Autodesk Fusion 360 part; units mm, degrees
(part 2 of 3)
sketch "Sketch15" plane through (0, 3, 0) normal (0, 1, 0) x (-1, 0, 0)
  line L0 (-66.9, 56.225) -> (-66.9, 85.865)
  line L1 (-66.9, 85.865) -> (-48.98, 85.865)
  line L2 (-48.98, 85.865) -> (-48.98, 56.225)
  line L3 (-48.98, 56.225) -> (-66.9, 56.225)
  line L4 (-83.08, 18.85) -> (0, 18.85)
  line L5 (0, 18.85) -> (0, 100)
  line L6 (0, 100) -> (-83.08, 100)
  line L7 (-83.08, 100) -> (-83.08, 18.85)
  line L8 (-38.05, 42.9) -> (-38.05, 56.9)
  line L9 (-38.05, 56.9) -> (-24.05, 56.9)
  line L10 (-24.05, 56.9) -> (-24.05, 42.9)
  line L11 (-24.05, 42.9) -> (-38.05, 42.9)
  line L12 (-19, 23.85) -> (-19, 37.85)
  line L13 (-19, 37.85) -> (-5, 37.85)
  line L14 (-5, 37.85) -> (-5, 23.85)
  line L15 (-5, 23.85) -> (-19, 23.85)
  line L16 (-19, 56.9) -> (-5, 56.9)
  line L17 (-5, 56.9) -> (-5, 42.9)
  line L18 (-5, 42.9) -> (-19, 42.9)
  line L19 (-19, 42.9) -> (-19, 56.9)
  line L20 (-38.05, 75.95) -> (-24.05, 75.95)
  line L21 (-24.05, 75.95) -> (-24.05, 61.95)
  line L22 (-24.05, 61.95) -> (-38.05, 61.95)
  line L23 (-38.05, 61.95) -> (-38.05, 75.95)
  line L24 (-19, 95) -> (-5, 95)
  line L25 (-5, 95) -> (-5, 81)
  line L26 (-5, 81) -> (-19, 81)
  line L27 (-19, 81) -> (-19, 95)
  line L28 (-38.05, 23.85) -> (-38.05, 37.85)
  line L29 (-38.05, 37.85) -> (-24.05, 37.85)
  line L30 (-24.05, 37.85) -> (-24.05, 23.85)
  line L31 (-24.05, 23.85) -> (-38.05, 23.85)
  line L32 (-19, 61.95) -> (-19, 75.95)
  line L33 (-19, 75.95) -> (-5, 75.95)
  line L34 (-5, 75.95) -> (-5, 61.95)
  line L35 (-5, 61.95) -> (-19, 61.95)
  line L36 (-38.05, 95) -> (-24.05, 95)
  line L37 (-24.05, 95) -> (-24.05, 81)
  line L38 (-24.05, 81) -> (-38.05, 81)
  line L39 (-38.05, 81) -> (-38.05, 95)
  circle A0 centre (-80.08, 97.0008) radius 1.5
  circle A1 centre (-2.9851, 97) radius 1.5
  circle A2 centre (-80.08, 21.85) radius 1.5
  circle A3 centre (-2.9679, 21.85) radius 1.5
  circle A4 centre (-60.755, 38.6) radius 4.5
extrude "Extrude26" add sketch "Sketch15" against normal blind 3 contours A0 | A1 | A2 | A3
sketch "Sketch16" plane through (0, 3, 0) normal (0, 1, 0) x (-1, 0, 0)
  line L0 (-66.9, 56.225) -> (-66.9, 85.865)
  line L1 (-66.9, 85.865) -> (-48.98, 85.865)
  line L2 (-48.98, 85.865) -> (-48.98, 56.225)
  line L3 (-48.98, 56.225) -> (-66.9, 56.225)
  line L4 (-83.08, 18.85) -> (0, 18.85)
  line L5 (0, 18.85) -> (0, 100)
  line L6 (0, 100) -> (-83.08, 100)
  line L7 (-83.08, 100) -> (-83.08, 18.85)
  line L8 (-38.05, 42.9) -> (-38.05, 56.9)
  line L9 (-38.05, 56.9) -> (-24.05, 56.9)
  line L10 (-24.05, 56.9) -> (-24.05, 42.9)
  line L11 (-24.05, 42.9) -> (-38.05, 42.9)
  line L12 (-19, 23.85) -> (-19, 37.85)
  line L13 (-19, 37.85) -> (-5, 37.85)
  line L14 (-5, 37.85) -> (-5, 23.85)
  line L15 (-5, 23.85) -> (-19, 23.85)
  line L16 (-19, 56.9) -> (-5, 56.9)
  line L17 (-5, 56.9) -> (-5, 42.9)
  line L18 (-5, 42.9) -> (-19, 42.9)
  line L19 (-19, 42.9) -> (-19, 56.9)
  line L20 (-38.05, 75.95) -> (-24.05, 75.95)
  line L21 (-24.05, 75.95) -> (-24.05, 61.95)
  line L22 (-24.05, 61.95) -> (-38.05, 61.95)
  line L23 (-38.05, 61.95) -> (-38.05, 75.95)
  line L24 (-19, 95) -> (-5, 95)
  line L25 (-5, 95) -> (-5, 81)
  line L26 (-5, 81) -> (-19, 81)
  line L27 (-19, 81) -> (-19, 95)
  line L28 (-38.05, 23.85) -> (-38.05, 37.85)
  line L29 (-38.05, 37.85) -> (-24.05, 37.85)
  line L30 (-24.05, 37.85) -> (-24.05, 23.85)
  line L31 (-24.05, 23.85) -> (-38.05, 23.85)
  line L32 (-19, 61.95) -> (-19, 75.95)
  line L33 (-19, 75.95) -> (-5, 75.95)
  line L34 (-5, 75.95) -> (-5, 61.95)
  line L35 (-5, 61.95) -> (-19, 61.95)
  line L36 (-38.05, 95) -> (-24.05, 95)
  line L37 (-24.05, 95) -> (-24.05, 81)
  line L38 (-24.05, 81) -> (-38.05, 81)
  line L39 (-38.05, 81) -> (-38.05, 95)
  circle A0 centre (-60.755, 38.6) radius 4.5
  line L40 (0, 21.368) -> (-2.5, 21.368)
  line L41 (-2.5, 21.368) -> (-2.5, 18.868)
  line L42 (-80.5906, 18.85) -> (-80.5906, 21.35)
  line L43 (-80.5906, 21.35) -> (-83.0906, 21.35)
  line L44 (-83.08, 97.4836) -> (-80.58, 97.4836)
  line L45 (-80.58, 97.4836) -> (-80.58, 99.9836)
  line L46 (0, 97.4763) -> (-2.5, 97.4763)
  line L47 (-2.5, 97.4763) -> (-2.5, 99.9763)
  circle A1 centre (-2.5, 97.4763) radius 1
  circle A2 centre (-80.58, 97.4836) radius 1
  circle A3 centre (-80.5906, 21.35) radius 1
  circle A4 centre (-2.5, 21.368) radius 1
  dimension "d162" = 2.5
  dimension "d163" = 2.5
  dimension "d164" = 2.5
  dimension "d165" = 2.5
  dimension "d166" = 2.5
  dimension "d167" = 2.5
  dimension "d168" = 2.5
  dimension "d169" = 2.5
  dimension "d170" = 2
  dimension "d171" = 2
  dimension "d172" = 2
  dimension "d173" = 2
  constraint coincident L5 L40.start
  constraint perpendicular L5 L40
  constraint perpendicular L40 L41
  constraint coincident L4 L42.start
  constraint perpendicular L4 L42
  constraint perpendicular L42 L43
  constraint coincident L7 L44.start
  constraint perpendicular L7 L44
  constraint perpendicular L44 L45
  constraint coincident L5 L46.start
  constraint perpendicular L5 L46
  constraint perpendicular L46 L47
  constraint coincident L46.end L47.start
  constraint coincident L44.end L45.start
  constraint coincident L42.end L43.start
  constraint coincident L40.end L41.start
  measures "d162" distance of L40.start L40.end
  measures "d163" distance of L40.end L41.end
  measures "d164" distance of L42.start L42.end
  measures "d165" distance of L42.end L43.end
  measures "d166" distance of L44.start L44.end
  measures "d167" distance of L44.end L45.end
  measures "d168" distance of L46.start L46.end
  measures "d169" distance of L46.end L47.end
  measures "d170" diameter of A1
  measures "d171" diameter of A2
  measures "d172" diameter of A3
  measures "d173" diameter of A4
extrude "Extrude27" cut sketch "Sketch16" against normal blind 5.5 contours L42 L43 A3 | L42 L43 A3 | L40 L41 A4 | L40 L41 A4 | L44 L45 A2 | L44 L45 A2 | L46 L47 A1 | L46 L47 A1
extrude "Extrude28" cut 4 faces at (44.9701, -4, 27.857) (77.0768, -4, 30.8265) (76.1742, -4, 90.9914) (44.34, -4, 90.7407) along direction (0, 1, 0) blind 0.5
extrude "Extrude29" cut 1 faces at (76.5447, 3, 58.3529) along direction (0, -1, 0) blind 1
extrude "Extrude30" cut 4 faces at (44.34, -3.5, 90.7407) (76.1742, -3.5, 90.9914) (77.0768, -3.5, 30.8265) (44.9701, -3.5, 27.857) along direction (0, 1, 0) blind 1
sketch "Sketch17" plane through (0, 2, 0) normal (0, 1, 0) x (-1, 0, 0)
  circle A0 centre (-80.5906, 21.35) radius 1
  circle A1 centre (-80.58, 97.4836) radius 1
  circle A2 centre (-2.5, 21.368) radius 1
  circle A3 centre (-2.5, 97.4763) radius 1
  line L0 (-66.9, 56.225) -> (-66.9, 85.865)
  line L1 (-66.9, 85.865) -> (-48.98, 85.865)
  line L2 (-48.98, 85.865) -> (-48.98, 56.225)
  line L3 (-48.98, 56.225) -> (-66.9, 56.225)
  line L4 (-83.08, 18.85) -> (0, 18.85)
  line L5 (0, 18.85) -> (0, 100)
  line L6 (0, 100) -> (-83.08, 100)
  line L7 (-83.08, 100) -> (-83.08, 18.85)
  line L8 (-38.05, 42.9) -> (-38.05, 56.9)
  line L9 (-38.05, 56.9) -> (-24.05, 56.9)
  line L10 (-24.05, 56.9) -> (-24.05, 42.9)
  line L11 (-24.05, 42.9) -> (-38.05, 42.9)
  line L12 (-19, 23.85) -> (-19, 37.85)
  line L13 (-19, 37.85) -> (-5, 37.85)
  line L14 (-5, 37.85) -> (-5, 23.85)
  line L15 (-5, 23.85) -> (-19, 23.85)
  line L16 (-19, 56.9) -> (-5, 56.9)
  line L17 (-5, 56.9) -> (-5, 42.9)
  line L18 (-5, 42.9) -> (-19, 42.9)
  line L19 (-19, 42.9) -> (-19, 56.9)
  line L20 (-38.05, 75.95) -> (-24.05, 75.95)
  line L21 (-24.05, 75.95) -> (-24.05, 61.95)
  line L22 (-24.05, 61.95) -> (-38.05, 61.95)
  line L23 (-38.05, 61.95) -> (-38.05, 75.95)
  line L24 (-19, 95) -> (-5, 95)
  line L25 (-5, 95) -> (-5, 81)
  line L26 (-5, 81) -> (-19, 81)
  line L27 (-19, 81) -> (-19, 95)
  line L28 (-38.05, 23.85) -> (-38.05, 37.85)
  line L29 (-38.05, 37.85) -> (-24.05, 37.85)
  line L30 (-24.05, 37.85) -> (-24.05, 23.85)
  line L31 (-24.05, 23.85) -> (-38.05, 23.85)
  line L32 (-19, 61.95) -> (-19, 75.95)
  line L33 (-19, 75.95) -> (-5, 75.95)
  line L34 (-5, 75.95) -> (-5, 61.95)
  line L35 (-5, 61.95) -> (-19, 61.95)
  line L36 (-38.05, 95) -> (-24.05, 95)
  line L37 (-24.05, 95) -> (-24.05, 81)
  line L38 (-24.05, 81) -> (-38.05, 81)
  line L39 (-38.05, 81) -> (-38.05, 95)
  circle A4 centre (-45.8889, 88.9935) radius 2
  circle A5 centre (-45.9348, 29.975) radius 2
  circle A6 centre (-75.1, 88.9) radius 2
  circle A7 centre (-74.9, 29.9) radius 2
  line L40 (-54.755, 44.6) -> (-54.755, 32.6)
  line L41 (-54.755, 32.6) -> (-66.755, 32.6)
  line L42 (-66.755, 32.6) -> (-66.755, 44.6)
  line L43 (-66.755, 44.6) -> (-54.755, 44.6)
extrude "Extrude31" add sketch "Sketch17" against normal blind 0.5 contours A4 | A5 | A6 | A7
sketch "Sketch18" plane through (0, 2, 0) normal (0, 1, 0) x (-1, 0, 0)
  circle A0 centre (-80.5906, 21.35) radius 1
  circle A1 centre (-80.58, 97.4836) radius 1
  circle A2 centre (-2.5, 21.368) radius 1
  circle A3 centre (-2.5, 97.4763) radius 1
  line L0 (-66.9, 56.225) -> (-66.9, 85.865)
  line L1 (-66.9, 85.865) -> (-48.98, 85.865)
  line L2 (-48.98, 85.865) -> (-48.98, 56.225)
  line L3 (-48.98, 56.225) -> (-66.9, 56.225)
  line L4 (-83.08, 18.85) -> (0, 18.85)
  line L5 (0, 18.85) -> (0, 100)
  line L6 (0, 100) -> (-83.08, 100)
  line L7 (-83.08, 100) -> (-83.08, 18.85)
  line L8 (-38.05, 42.9) -> (-38.05, 56.9)
  line L9 (-38.05, 56.9) -> (-24.05, 56.9)
  line L10 (-24.05, 56.9) -> (-24.05, 42.9)
  line L11 (-24.05, 42.9) -> (-38.05, 42.9)
  line L12 (-19, 23.85) -> (-19, 37.85)
  line L13 (-19, 37.85) -> (-5, 37.85)
  line L14 (-5, 37.85) -> (-5, 23.85)
  line L15 (-5, 23.85) -> (-19, 23.85)
  line L16 (-19, 56.9) -> (-5, 56.9)
  line L17 (-5, 56.9) -> (-5, 42.9)
  line L18 (-5, 42.9) -> (-19, 42.9)
  line L19 (-19, 42.9) -> (-19, 56.9)
  line L20 (-38.05, 75.95) -> (-24.05, 75.95)
  line L21 (-24.05, 75.95) -> (-24.05, 61.95)
  line L22 (-24.05, 61.95) -> (-38.05, 61.95)
  line L23 (-38.05, 61.95) -> (-38.05, 75.95)
  line L24 (-19, 95) -> (-5, 95)
  line L25 (-5, 95) -> (-5, 81)
  line L26 (-5, 81) -> (-19, 81)
  line L27 (-19, 81) -> (-19, 95)
  line L28 (-38.05, 23.85) -> (-38.05, 37.85)
  line L29 (-38.05, 37.85) -> (-24.05, 37.85)
  line L30 (-24.05, 37.85) -> (-24.05, 23.85)
  line L31 (-24.05, 23.85) -> (-38.05, 23.85)
  line L32 (-19, 61.95) -> (-19, 75.95)
  line L33 (-19, 75.95) -> (-5, 75.95)
  line L34 (-5, 75.95) -> (-5, 61.95)
  line L35 (-5, 61.95) -> (-19, 61.95)
  line L36 (-38.05, 95) -> (-24.05, 95)
  line L37 (-24.05, 95) -> (-24.05, 81)
  line L38 (-24.05, 81) -> (-38.05, 81)
  line L39 (-38.05, 81) -> (-38.05, 95)
  line L40 (-54.755, 44.6) -> (-54.755, 32.6)
  line L41 (-54.755, 32.6) -> (-66.755, 32.6)
  line L42 (-66.755, 32.6) -> (-66.755, 44.6)
  line L43 (-66.755, 44.6) -> (-54.755, 44.6)
extrude "Extrude32" add sketch "Sketch18" against normal blind 0.5 contours L40 L41 L42 L43
sketch "Sketch19" plane through (0, 1.5, 0) normal (0, -1, 0) x (1, 0, 0)
  line L0 (66.755, 32.6) -> (66.755, 44.6)
  line L1 (66.755, 44.6) -> (54.755, 44.6)
  line L2 (54.755, 44.6) -> (54.755, 32.6)
  line L3 (54.755, 32.6) -> (66.755, 32.6)
  circle A0 centre (60.7672, 38.6189) radius 6
  dimension "d186" = 12
  measures "d186" diameter of A0
extrude "Extrude33" cut sketch "Sketch19" against normal blind 1 contours L0 L1 A0 picked at (62.3334, 39.4206)
sketch "Sketch20" plane through (0, 0, 0) normal (0, -1, 0) x (1, 0, 0)
  line L0 (66.9, 85.865) -> (66.9, 56.225)
  line L1 (66.9, 56.225) -> (48.98, 56.225)
  line L2 (48.98, 56.225) -> (48.98, 85.7386)
  arc A0 (49.1082, 85.865) -> (48.98, 85.7386) centre (45.8848, 89.005) ccw
  line L3 (49.1082, 85.865) -> (66.9, 85.865)
  circle A1 centre (75.1296, 88.925) radius 4.5
  circle A2 centre (45.9348, 29.975) radius 4.5
  line L4 (83.08, 100) -> (0, 100)
  line L5 (0, 100) -> (0, 18.85)
  line L6 (0, 18.85) -> (83.08, 18.85)
  line L7 (83.08, 18.85) -> (83.08, 100)
  line L8 (24.05, 95) -> (38.05, 95)
  line L9 (38.05, 95) -> (38.05, 81)
  line L10 (38.05, 81) -> (24.05, 81)
  line L11 (24.05, 81) -> (24.05, 95)
  line L12 (19, 75.95) -> (19, 61.95)
  line L13 (19, 61.95) -> (5, 61.95)
  line L14 (5, 61.95) -> (5, 75.95)
  line L15 (5, 75.95) -> (19, 75.95)
  line L16 (38.05, 37.85) -> (38.05, 23.85)
  line L17 (38.05, 23.85) -> (24.05, 23.85)
  line L18 (24.05, 23.85) -> (24.05, 37.85)
  line L19 (24.05, 37.85) -> (38.05, 37.85)
  line L20 (5, 95) -> (19, 95)
  line L21 (19, 95) -> (19, 81)
  line L22 (19, 81) -> (5, 81)
  line L23 (5, 81) -> (5, 95)
  line L24 (24.05, 75.95) -> (38.05, 75.95)
  line L25 (38.05, 75.95) -> (38.05, 61.95)
  line L26 (38.05, 61.95) -> (24.05, 61.95)
  line L27 (24.05, 61.95) -> (24.05, 75.95)
  line L28 (5, 56.9) -> (19, 56.9)
  line L29 (19, 56.9) -> (19, 42.9)
  line L30 (19, 42.9) -> (5, 42.9)
  line L31 (5, 42.9) -> (5, 56.9)
  line L32 (19, 37.85) -> (19, 23.85)
  line L33 (19, 23.85) -> (5, 23.85)
  line L34 (5, 23.85) -> (5, 37.85)
  line L35 (5, 37.85) -> (19, 37.85)
  line L36 (38.05, 56.9) -> (38.05, 42.9)
  line L37 (38.05, 42.9) -> (24.05, 42.9)
  line L38 (24.05, 42.9) -> (24.05, 56.9)
  line L39 (24.05, 56.9) -> (38.05, 56.9)
  line L40 (54.755, 44.6) -> (66.755, 44.6)
  line L41 (66.755, 44.6) -> (66.755, 32.6)
  line L42 (66.755, 32.6) -> (54.755, 32.6)
  line L43 (54.755, 32.6) -> (54.755, 44.6)
  circle A3 centre (74.9435, 29.945) radius 4.5
  circle A4 centre (2.5, 97.4763) radius 1
  circle A5 centre (2.5, 21.368) radius 1
  circle A6 centre (80.58, 97.4836) radius 1
  circle A7 centre (80.5906, 21.35) radius 1
extrude "Extrude34" add sketch "Sketch20" against normal blind 2 contours A4 | A5 | A6 | A7
sketch "Sketch21" plane through (0, 0, 0) normal (0, -1, 0) x (1, 0, 0)
  line L0 (66.9, 85.865) -> (66.9, 56.225)
  line L1 (66.9, 56.225) -> (48.98, 56.225)
  line L2 (48.98, 56.225) -> (48.98, 85.7386)
  arc A0 (49.1082, 85.865) -> (48.98, 85.7386) centre (45.8848, 89.005) ccw
  line L3 (49.1082, 85.865) -> (66.9, 85.865)
  circle A1 centre (75.1296, 88.925) radius 4.5
  circle A2 centre (45.9348, 29.975) radius 4.5
  line L4 (83.08, 100) -> (0, 100)
  line L5 (0, 100) -> (0, 18.85)
  line L6 (0, 18.85) -> (83.08, 18.85)
  line L7 (83.08, 18.85) -> (83.08, 100)
  line L8 (24.05, 95) -> (38.05, 95)
  line L9 (38.05, 95) -> (38.05, 81)
  line L10 (38.05, 81) -> (24.05, 81)
  line L11 (24.05, 81) -> (24.05, 95)
  line L12 (19, 75.95) -> (19, 61.95)
  line L13 (19, 61.95) -> (5, 61.95)
  line L14 (5, 61.95) -> (5, 75.95)
  line L15 (5, 75.95) -> (19, 75.95)
  line L16 (38.05, 37.85) -> (38.05, 23.85)
  line L17 (38.05, 23.85) -> (24.05, 23.85)
  line L18 (24.05, 23.85) -> (24.05, 37.85)
  line L19 (24.05, 37.85) -> (38.05, 37.85)
  line L20 (5, 95) -> (19, 95)
  line L21 (19, 95) -> (19, 81)
  line L22 (19, 81) -> (5, 81)
  line L23 (5, 81) -> (5, 95)
  line L24 (24.05, 75.95) -> (38.05, 75.95)
  line L25 (38.05, 75.95) -> (38.05, 61.95)
  line L26 (38.05, 61.95) -> (24.05, 61.95)
  line L27 (24.05, 61.95) -> (24.05, 75.95)
  line L28 (5, 56.9) -> (19, 56.9)
  line L29 (19, 56.9) -> (19, 42.9)
  line L30 (19, 42.9) -> (5, 42.9)
  line L31 (5, 42.9) -> (5, 56.9)
  line L32 (19, 37.85) -> (19, 23.85)
  line L33 (19, 23.85) -> (5, 23.85)
  line L34 (5, 23.85) -> (5, 37.85)
  line L35 (5, 37.85) -> (19, 37.85)
  line L36 (38.05, 56.9) -> (38.05, 42.9)
  line L37 (38.05, 42.9) -> (24.05, 42.9)
  line L38 (24.05, 42.9) -> (24.05, 56.9)
  line L39 (24.05, 56.9) -> (38.05, 56.9)
  line L40 (54.755, 44.6) -> (66.755, 44.6)
  line L41 (66.755, 44.6) -> (66.755, 32.6)
  line L42 (66.755, 32.6) -> (54.755, 32.6)
  line L43 (54.755, 32.6) -> (54.755, 44.6)
  circle A3 centre (74.9435, 29.945) radius 4.5
  circle A4 centre (3.9673, 22.8373) radius 4
  circle A5 centre (3.9951, 96.0403) radius 4
  circle A6 centre (79.0997, 96.034) radius 4
  circle A7 centre (79.1068, 22.8281) radius 4
  dimension "d191" = 8
  dimension "d192" = 5.625
  dimension "d193" = 8
  dimension "d194" = 8
  dimension "d195" = 8
  measures "d191" diameter of A4
  measures "d192" distance of L4.end A5.centre
  measures "d193" diameter of A5
  measures "d194" diameter of A6
  measures "d195" diameter of A7
extrude "Extrude35" cut sketch "Sketch21" against normal blind 3 contours L4 L7 A6 | L6 L7 A7 | L4 L5 A5 | L5 L6 A4
extrude "Extrude36" cut 2 faces at (65.3995, 1.5, 43.6074) (55.9645, 1.5, 33.7699) along direction (0, 1, 0) blind 0.1
sketch "Sketch22" plane through (0, 0, 0) normal (0, -1, 0) x (1, 0, 0)
  arc A0 (0, 22.3271) -> (3.6486, 18.85) centre (3.9673, 22.8373) ccw
  line L0 (3.6486, 18.85) -> (79.525, 18.85)
  arc A1 (79.525, 18.85) -> (83.08, 22.3661) centre (79.1068, 22.8281) ccw
  line L1 (83.08, 22.3661) -> (83.08, 96.4304)
  arc A2 (83.08, 96.4304) -> (79.62, 100) centre (79.0997, 96.034) ccw
  line L2 (79.62, 100) -> (3.429, 100)
  arc A3 (3.429, 100) -> (0, 96.2373) centre (3.9951, 96.0403) ccw
  line L3 (0, 96.2373) -> (0, 22.3271)
  circle A4 centre (74.9435, 29.945) radius 4.5
  line L4 (54.755, 44.6) -> (66.755, 44.6)
  line L5 (66.755, 44.6) -> (66.755, 32.6)
  line L6 (66.755, 32.6) -> (54.755, 32.6)
  line L7 (54.755, 32.6) -> (54.755, 44.6)
  line L8 (38.05, 56.9) -> (38.05, 42.9)
  line L9 (38.05, 42.9) -> (24.05, 42.9)
  line L10 (24.05, 42.9) -> (24.05, 56.9)
  line L11 (24.05, 56.9) -> (38.05, 56.9)
  line L12 (19, 37.85) -> (19, 23.85)
  line L13 (19, 23.85) -> (5, 23.85)
  line L14 (5, 23.85) -> (5, 37.85)
  line L15 (5, 37.85) -> (19, 37.85)
  line L16 (5, 56.9) -> (19, 56.9)
  line L17 (19, 56.9) -> (19, 42.9)
  line L18 (19, 42.9) -> (5, 42.9)
  line L19 (5, 42.9) -> (5, 56.9)
  line L20 (24.05, 75.95) -> (38.05, 75.95)
  line L21 (38.05, 75.95) -> (38.05, 61.95)
  line L22 (38.05, 61.95) -> (24.05, 61.95)
  line L23 (24.05, 61.95) -> (24.05, 75.95)
  line L24 (5, 95) -> (19, 95)
  line L25 (19, 95) -> (19, 81)
  line L26 (19, 81) -> (5, 81)
  line L27 (5, 81) -> (5, 95)
  line L28 (38.05, 37.85) -> (38.05, 23.85)
  line L29 (38.05, 23.85) -> (24.05, 23.85)
  line L30 (24.05, 23.85) -> (24.05, 37.85)
  line L31 (24.05, 37.85) -> (38.05, 37.85)
  line L32 (19, 75.95) -> (19, 61.95)
  line L33 (19, 61.95) -> (5, 61.95)
  line L34 (5, 61.95) -> (5, 75.95)
  line L35 (5, 75.95) -> (19, 75.95)
  line L36 (24.05, 95) -> (38.05, 95)
  line L37 (38.05, 95) -> (38.05, 81)
  line L38 (38.05, 81) -> (24.05, 81)
  line L39 (24.05, 81) -> (24.05, 95)
  circle A5 centre (45.9348, 29.975) radius 4.5
  circle A6 centre (75.1296, 88.925) radius 4.5
  line L40 (66.9, 85.865) -> (66.9, 56.225)
  line L41 (66.9, 56.225) -> (48.98, 56.225)
  line L42 (48.98, 56.225) -> (48.98, 85.7386)
  arc A7 (49.1082, 85.865) -> (48.98, 85.7386) centre (45.8848, 89.005) ccw
  line L43 (49.1082, 85.865) -> (66.9, 85.865)
  circle A8 centre (3, 97) radius 1.75
  circle A9 centre (3, 97) radius 1
  line L44 (3, 97) -> (3, 100)
  line L45 (3, 97) -> (0, 97)
  line L46 (80.0899, 100) -> (80.0899, 97)
  line L47 (80.0899, 97) -> (83.0899, 97)
  circle A10 centre (80.0899, 97) radius 1
  line L48 (83.0763, 21.8589) -> (80.0763, 21.8589)
  line L49 (80.0763, 21.8589) -> (80.0763, 18.8589)
  circle A11 centre (80.0763, 21.8589) radius 1
  line L50 (-0.0037, 21.8321) -> (2.9963, 21.8321)
  line L51 (2.9963, 21.8321) -> (2.9963, 18.8321)
  circle A12 centre (2.9963, 21.8321) radius 1
  dimension "d200" = 3.5
  dimension "d201" = 2
  dimension "d202" = 3
  dimension "d203" = 3
  dimension "d204" = 2
  dimension "d205" = 3
  dimension "d206" = 3
  dimension "d207" = 2
  dimension "d208" = 3
  dimension "d209" = 3
  dimension "d210" = 2
  constraint concentric A8 A9
  constraint coincident A8.centre A9.centre
  constraint vertical L44
  constraint horizontal L45
  constraint vertical L46
  constraint perpendicular L1 L47
  constraint coincident L46.end L47.start
  constraint horizontal L48
  constraint perpendicular L48 L49
  constraint coincident L48.end L49.start
  constraint horizontal L50
  constraint perpendicular L50 L51
  constraint coincident L50.end L51.start
  measures "d200" diameter of A8
  measures "d201" diameter of A9
  measures "d202" distance of L46.start L46.end
  measures "d203" distance of L46.end L47.end
  measures "d204" diameter of A10
  measures "d205" distance of L48.start L48.end
  measures "d206" distance of L48.end L49.end
  measures "d207" diameter of A11
  measures "d208" distance of L50.start L50.end
  measures "d209" distance of L50.end L51.end
  measures "d210" diameter of A12
extrude "Extrude37" cut sketch "Sketch22" against normal blind 7 contours L50 L51 A12 | L50 L51 A12 | A9 L44 L45 | A9 L44 L45 | L48 L49 A11 | L48 L49 A11 | L46 L47 A10 | L46 L47 A10
sketch "Sketch23" plane through (0, 0, 0) normal (0, -1, 0) x (1, 0, 0)
  line L0 (66.9, 85.865) -> (66.9, 56.225)
  line L1 (66.9, 56.225) -> (48.98, 56.225)
  line L2 (48.98, 56.225) -> (48.98, 85.7386)
  arc A0 (49.1082, 85.865) -> (48.98, 85.7386) centre (45.8848, 89.005) ccw
  line L3 (49.1082, 85.865) -> (66.9, 85.865)
  circle A1 centre (75.1296, 88.925) radius 4.5
  circle A2 centre (45.9348, 29.975) radius 4.5
  line L4 (24.05, 95) -> (38.05, 95)
  line L5 (38.05, 95) -> (38.05, 81)
  line L6 (38.05, 81) -> (24.05, 81)
  line L7 (24.05, 81) -> (24.05, 95)
  line L8 (19, 75.95) -> (19, 61.95)
  line L9 (19, 61.95) -> (5, 61.95)
  line L10 (5, 61.95) -> (5, 75.95)
  line L11 (5, 75.95) -> (19, 75.95)
  line L12 (38.05, 37.85) -> (38.05, 23.85)
  line L13 (38.05, 23.85) -> (24.05, 23.85)
  line L14 (24.05, 23.85) -> (24.05, 37.85)
  line L15 (24.05, 37.85) -> (38.05, 37.85)
  line L16 (5, 95) -> (19, 95)
  line L17 (19, 95) -> (19, 81)
  line L18 (19, 81) -> (5, 81)
  line L19 (5, 81) -> (5, 95)
  line L20 (24.05, 75.95) -> (38.05, 75.95)
  line L21 (38.05, 75.95) -> (38.05, 61.95)
  line L22 (38.05, 61.95) -> (24.05, 61.95)
  line L23 (24.05, 61.95) -> (24.05, 75.95)
  line L24 (5, 56.9) -> (19, 56.9)
  line L25 (19, 56.9) -> (19, 42.9)
  line L26 (19, 42.9) -> (5, 42.9)
  line L27 (5, 42.9) -> (5, 56.9)
  line L28 (19, 37.85) -> (19, 23.85)
  line L29 (19, 23.85) -> (5, 23.85)
  line L30 (5, 23.85) -> (5, 37.85)
  line L31 (5, 37.85) -> (19, 37.85)
  line L32 (38.05, 56.9) -> (38.05, 42.9)
  line L33 (38.05, 42.9) -> (24.05, 42.9)
  line L34 (24.05, 42.9) -> (24.05, 56.9)
  line L35 (24.05, 56.9) -> (38.05, 56.9)
  line L36 (54.755, 44.6) -> (66.755, 44.6)
  line L37 (66.755, 44.6) -> (66.755, 32.6)
  line L38 (66.755, 32.6) -> (54.755, 32.6)
  line L39 (54.755, 32.6) -> (54.755, 44.6)
  circle A3 centre (74.9435, 29.945) radius 4.5
  arc A4 (0, 22.3271) -> (3.6486, 18.85) centre (3.9673, 22.8373) ccw
  line L40 (3.6486, 18.85) -> (79.525, 18.85)
  arc A5 (79.525, 18.85) -> (83.08, 22.3661) centre (79.1068, 22.8281) ccw
  line L41 (83.08, 22.3661) -> (83.08, 96.4304)
  arc A6 (83.08, 96.4304) -> (79.62, 100) centre (79.0997, 96.034) ccw
  line L42 (79.62, 100) -> (3.429, 100)
  arc A7 (3.429, 100) -> (0, 96.2373) centre (3.9951, 96.0403) ccw
  line L43 (0, 96.2373) -> (0, 22.3271)
  circle A8 centre (80.0763, 21.8589) radius 1
  circle A9 centre (2.9963, 21.8321) radius 1
  circle A10 centre (80.0899, 97) radius 1
  circle A11 centre (3, 97) radius 1
sketch "Sketch24" plane through (0, 2, 0) normal (0, 1, 0) x (-1, 0, 0)
  line L0 (-38.05, 95) -> (-24.05, 95)
  line L1 (-24.05, 95) -> (-24.05, 81)
  line L2 (-24.05, 81) -> (-38.05, 81)
  line L3 (-38.05, 81) -> (-38.05, 95)
  line L4 (-19, 61.95) -> (-19, 75.95)
  line L5 (-19, 75.95) -> (-5, 75.95)
  line L6 (-5, 75.95) -> (-5, 61.95)
  line L7 (-5, 61.95) -> (-19, 61.95)
  line L8 (-38.05, 23.85) -> (-38.05, 37.85)
  line L9 (-38.05, 37.85) -> (-24.05, 37.85)
  line L10 (-24.05, 37.85) -> (-24.05, 23.85)
  line L11 (-24.05, 23.85) -> (-38.05, 23.85)
  line L12 (-19, 95) -> (-5, 95)
  line L13 (-5, 95) -> (-5, 81)
  line L14 (-5, 81) -> (-19, 81)
  line L15 (-19, 81) -> (-19, 95)
  line L16 (-38.05, 75.95) -> (-24.05, 75.95)
  line L17 (-24.05, 75.95) -> (-24.05, 61.95)
  line L18 (-24.05, 61.95) -> (-38.05, 61.95)
  line L19 (-38.05, 61.95) -> (-38.05, 75.95)
  line L20 (-19, 56.9) -> (-5, 56.9)
  line L21 (-5, 56.9) -> (-5, 42.9)
  line L22 (-5, 42.9) -> (-19, 42.9)
  line L23 (-19, 42.9) -> (-19, 56.9)
  line L24 (-19, 23.85) -> (-19, 37.85)
  line L25 (-19, 37.85) -> (-5, 37.85)
  line L26 (-5, 37.85) -> (-5, 23.85)
  line L27 (-5, 23.85) -> (-19, 23.85)
  line L28 (-38.05, 42.9) -> (-38.05, 56.9)
  line L29 (-38.05, 56.9) -> (-24.05, 56.9)
  line L30 (-24.05, 56.9) -> (-24.05, 42.9)
  line L31 (-24.05, 42.9) -> (-38.05, 42.9)
  line L32 (-66.9, 56.225) -> (-66.9, 85.865)
  line L33 (-66.9, 85.865) -> (-48.98, 85.865)
  line L34 (-48.98, 85.865) -> (-48.98, 56.225)
  line L35 (-48.98, 56.225) -> (-66.9, 56.225)
  arc A0 (-61.2435, 44.6) -> (-66.755, 39.0018) centre (-60.7672, 38.6189) ccw
  line L36 (-61.2435, 44.6) -> (-60.2909, 44.6)
  arc A1 (-66.755, 38.2361) -> (-60.2909, 44.6) centre (-60.7672, 38.6189) ccw
  line L37 (-66.755, 38.2361) -> (-66.755, 39.0018)
  arc A2 (-3.6486, 18.85) -> (0, 22.3271) centre (-3.9673, 22.8373) ccw
  line L38 (0, 22.3271) -> (0, 96.2373)
  arc A3 (0, 96.2373) -> (-3.429, 100) centre (-3.9951, 96.0403) ccw
  line L39 (-3.429, 100) -> (-79.62, 100)
  arc A4 (-79.62, 100) -> (-83.08, 96.4304) centre (-79.0997, 96.034) ccw
  line L40 (-83.08, 96.4304) -> (-83.08, 22.3661)
  arc A5 (-83.08, 22.3661) -> (-79.525, 18.85) centre (-79.1068, 22.8281) ccw
  line L41 (-79.525, 18.85) -> (-3.6486, 18.85)
  circle A6 centre (-80.0763, 21.8589) radius 1
  circle A7 centre (-2.9963, 21.8321) radius 1
  circle A8 centre (-80.0899, 97) radius 1
  circle A9 centre (-3, 97) radius 1
  line L42 (-83.08, 18.85) -> (0, 18.85)
  line L43 (0, 18.85) -> (0, 100)
  line L44 (0, 100) -> (-83.08, 100)
  line L45 (-83.08, 100) -> (-83.08, 18.85)
  constraint horizontal L42
  constraint vertical L43
  constraint horizontal L44
  constraint vertical L45
delete_face "DeleteFace5" 1 faces at (81.6049, 1.3333, 99.1523)
delete_face "DeleteFace6" 1 faces at (81.7888, 1.3333, 19.8605)
extrude "Extrude38" cut 1 faces at (83.08, 0.6667, 72.95) along direction (-1, 0, 0) blind 1.93
sketch "Sketch25" plane through (0, 0, 0) normal (0, -1, 0) x (1, 0, 0)
  line L0 (81.15, 18.85) -> (81.15, 100)
  line L1 (81.15, 100) -> (3.429, 100)
  arc A0 (3.429, 100) -> (0, 96.2373) centre (3.9951, 96.0403) ccw
  line L2 (0, 96.2373) -> (0, 22.3271)
  arc A1 (0, 22.3271) -> (3.6486, 18.85) centre (3.9673, 22.8373) ccw
  line L3 (3.6486, 18.85) -> (81.15, 18.85)
  circle A2 centre (3, 97) radius 1
  circle A3 centre (80.0899, 97) radius 1
  circle A4 centre (2.9963, 21.8321) radius 1
  circle A5 centre (80.0763, 21.8589) radius 1
  circle A6 centre (74.9435, 29.945) radius 4.5
  line L4 (54.755, 44.6) -> (66.755, 44.6)
  line L5 (66.755, 44.6) -> (66.755, 32.6)
  line L6 (66.755, 32.6) -> (54.755, 32.6)
  line L7 (54.755, 32.6) -> (54.755, 44.6)
  line L8 (38.05, 56.9) -> (38.05, 42.9)
  line L9 (38.05, 42.9) -> (24.05, 42.9)
  line L10 (24.05, 42.9) -> (24.05, 56.9)
  line L11 (24.05, 56.9) -> (38.05, 56.9)
  line L12 (19, 37.85) -> (19, 23.85)
  line L13 (19, 23.85) -> (5, 23.85)
  line L14 (5, 23.85) -> (5, 37.85)
  line L15 (5, 37.85) -> (19, 37.85)
  line L16 (5, 56.9) -> (19, 56.9)
  line L17 (19, 56.9) -> (19, 42.9)
  line L18 (19, 42.9) -> (5, 42.9)
  line L19 (5, 42.9) -> (5, 56.9)
  line L20 (24.05, 75.95) -> (38.05, 75.95)
  line L21 (38.05, 75.95) -> (38.05, 61.95)
  line L22 (38.05, 61.95) -> (24.05, 61.95)
  line L23 (24.05, 61.95) -> (24.05, 75.95)
  line L24 (5, 95) -> (19, 95)
  line L25 (19, 95) -> (19, 81)
  line L26 (19, 81) -> (5, 81)
  line L27 (5, 81) -> (5, 95)
  line L28 (38.05, 37.85) -> (38.05, 23.85)
  line L29 (38.05, 23.85) -> (24.05, 23.85)
  line L30 (24.05, 23.85) -> (24.05, 37.85)
  line L31 (24.05, 37.85) -> (38.05, 37.85)
  line L32 (19, 75.95) -> (19, 61.95)
  line L33 (19, 61.95) -> (5, 61.95)
  line L34 (5, 61.95) -> (5, 75.95)
  line L35 (5, 75.95) -> (19, 75.95)
  line L36 (24.05, 95) -> (38.05, 95)
  line L37 (38.05, 95) -> (38.05, 81)
  line L38 (38.05, 81) -> (24.05, 81)
  line L39 (24.05, 81) -> (24.05, 95)
  circle A7 centre (45.9348, 29.975) radius 4.5
  circle A8 centre (75.1296, 88.925) radius 4.5
  line L40 (66.9, 85.865) -> (66.9, 56.225)
  line L41 (66.9, 56.225) -> (48.98, 56.225)
  line L42 (48.98, 56.225) -> (48.98, 85.7386)
  arc A9 (49.1082, 85.865) -> (48.98, 85.7386) centre (45.8848, 89.005) ccw
  line L43 (49.1082, 85.865) -> (66.9, 85.865)
extrude "Extrude39" add sketch "Sketch25" against normal blind 2 contours A3 | A5
sketch "Sketch26" plane through (0, 0, 0) normal (0, -1, 0) x (1, 0, 0)
  line L0 (81.15, 18.85) -> (81.15, 100)
  line L1 (81.15, 100) -> (3.429, 100)
  arc A0 (3.429, 100) -> (0, 96.2373) centre (3.9951, 96.0403) ccw
  line L2 (0, 96.2373) -> (0, 22.3271)
  arc A1 (0, 22.3271) -> (3.6486, 18.85) centre (3.9673, 22.8373) ccw
  line L3 (3.6486, 18.85) -> (81.15, 18.85)
  circle A2 centre (3, 97) radius 1
  circle A3 centre (2.9963, 21.8321) radius 1
  circle A4 centre (74.9435, 29.945) radius 4.5
  line L4 (54.755, 44.6) -> (66.755, 44.6)
  line L5 (66.755, 44.6) -> (66.755, 32.6)
  line L6 (66.755, 32.6) -> (54.755, 32.6)
  line L7 (54.755, 32.6) -> (54.755, 44.6)
  line L8 (38.05, 56.9) -> (38.05, 42.9)
  line L9 (38.05, 42.9) -> (24.05, 42.9)
  line L10 (24.05, 42.9) -> (24.05, 56.9)
  line L11 (24.05, 56.9) -> (38.05, 56.9)
  line L12 (19, 37.85) -> (19, 23.85)
  line L13 (19, 23.85) -> (5, 23.85)
  line L14 (5, 23.85) -> (5, 37.85)
  line L15 (5, 37.85) -> (19, 37.85)
  line L16 (5, 56.9) -> (19, 56.9)
  line L17 (19, 56.9) -> (19, 42.9)
  line L18 (19, 42.9) -> (5, 42.9)
  line L19 (5, 42.9) -> (5, 56.9)
  line L20 (24.05, 75.95) -> (38.05, 75.95)
  line L21 (38.05, 75.95) -> (38.05, 61.95)
  line L22 (38.05, 61.95) -> (24.05, 61.95)
  line L23 (24.05, 61.95) -> (24.05, 75.95)
  line L24 (5, 95) -> (19, 95)
  line L25 (19, 95) -> (19, 81)
  line L26 (19, 81) -> (5, 81)
  line L27 (5, 81) -> (5, 95)
  line L28 (38.05, 37.85) -> (38.05, 23.85)
  line L29 (38.05, 23.85) -> (24.05, 23.85)
  line L30 (24.05, 23.85) -> (24.05, 37.85)
  line L31 (24.05, 37.85) -> (38.05, 37.85)
  line L32 (19, 75.95) -> (19, 61.95)
  line L33 (19, 61.95) -> (5, 61.95)
  line L34 (5, 61.95) -> (5, 75.95)
  line L35 (5, 75.95) -> (19, 75.95)
  line L36 (24.05, 95) -> (38.05, 95)
  line L37 (38.05, 95) -> (38.05, 81)
  line L38 (38.05, 81) -> (24.05, 81)
  line L39 (24.05, 81) -> (24.05, 95)
  circle A5 centre (45.9348, 29.975) radius 4.5
  circle A6 centre (75.1296, 88.925) radius 4.5
  line L40 (66.9, 85.865) -> (66.9, 56.225)
  line L41 (66.9, 56.225) -> (48.98, 56.225)
  line L42 (48.98, 56.225) -> (48.98, 85.7386)
  arc A7 (49.1082, 85.865) -> (48.98, 85.7386) centre (45.8848, 89.005) ccw
  line L43 (49.1082, 85.865) -> (66.9, 85.865)
  line L44 (78.1473, 18.85) -> (78.1473, 21.85)
  line L45 (78.1473, 21.85) -> (81.1473, 21.85)
  circle A8 centre (78.1473, 21.85) radius 1
  line L46 (81.15, 97.0036) -> (78.15, 97.0036)
  line L47 (78.15, 97.0036) -> (78.15, 100.0036)
  circle A9 centre (78.15, 97.0036) radius 1
  line L48 (81.15, 100) -> (81.15, 96)
  line L49 (81.15, 96) -> (77.15, 96)
  circle A10 centre (77.15, 96) radius 4
  line L50 (81.15, 18.85) -> (77.15, 18.85)
  line L51 (77.15, 18.85) -> (77.15, 22.85)
  circle A11 centre (77.15, 22.85) radius 4
  dimension "d217" = 3
  dimension "d218" = 3
  dimension "d219" = 2
  dimension "d220" = 3
  dimension "d221" = 3
  dimension "d222" = 2
  dimension "d223" = 4
  dimension "d224" = 4
  dimension "d225" = 8
  dimension "d226" = 4
  dimension "d227" = 4
  dimension "d228" = 8
  constraint coincident L3 L44.start
  constraint perpendicular L3 L44
  constraint perpendicular L44 L45
  constraint coincident L44.end L45.start
  constraint coincident L0 L46.start
  constraint perpendicular L0 L46
  constraint perpendicular L46 L47
  constraint coincident L46.end L47.start
  constraint coincident L0.end L1.start
  constraint perpendicular L1 L48
  constraint perpendicular L0 L49
  constraint coincident L49.end A10.centre
  constraint coincident L0.start L3.end
  constraint perpendicular L0 L50
  constraint perpendicular L3 L51
  constraint coincident L51.end A11.centre
  measures "d217" distance of L44.start L44.end
  measures "d218" distance of L44.end L45.end
  measures "d219" diameter of A8
  measures "d220" distance of L46.start L46.end
  measures "d221" distance of L46.end L47.end
  measures "d222" diameter of A9
  measures "d223" distance of L0.end L48.end
  measures "d224" distance of L48.end L49.end
  measures "d225" diameter of A10
  measures "d226" distance of L0.start L50.end
  measures "d227" distance of L50.end L51.end
  measures "d228" diameter of A11
extrude "Extrude40" cut sketch "Sketch26" against normal blind 5.5 contours L0 L3 L44 L50 A11 | L3 L44 L50 A11 | L0 L46 L48 A10 | L0 L1 L46 L47 L48 A10 | L44 L45 A8 | L44 L45 A8 L51 | L46 L47 A9 | L46 L47 A9 | L1 L47 A10
delete_face "DeleteFace7" 1 faces at (81.1455, 1.3333, 22.6597)
delete_face "DeleteFace8" 1 faces at (3.4678, 1.3333, 18.8686)
delete_face "DeleteFace9" 1 faces at (0.8037, 1.3333, 98.4516)
delete_face "DeleteFace10" 1 faces at (81.0372, 1.3333, 96.943)
extrude "Extrude41" add 1 faces at (54.1, 0.6667, 18.85) along direction (0, 0, -1) blind 0.965
extrude "Extrude42" add 1 faces at (27.05, 0.6667, 100) along direction (0, 0, 1) blind 0.965
sketch "Sketch27" plane through (0, 2, 0) normal (0, 1, 0) x (-1, 0, 0)
  line L0 (-81.15, 100.965) -> (-81.15, 17.885)
  line L1 (-81.15, 17.885) -> (0, 17.885)
  line L2 (0, 17.885) -> (0, 100.965)
  line L3 (0, 100.965) -> (-81.15, 100.965)
  line L4 (-38.05, 95) -> (-24.05, 95)
  line L5 (-24.05, 95) -> (-24.05, 81)
  line L6 (-24.05, 81) -> (-38.05, 81)
  line L7 (-38.05, 81) -> (-38.05, 95)
  line L8 (-19, 61.95) -> (-19, 75.95)
  line L9 (-19, 75.95) -> (-5, 75.95)
  line L10 (-5, 75.95) -> (-5, 61.95)
  line L11 (-5, 61.95) -> (-19, 61.95)
  line L12 (-38.05, 23.85) -> (-38.05, 37.85)
  line L13 (-38.05, 37.85) -> (-24.05, 37.85)
  line L14 (-24.05, 37.85) -> (-24.05, 23.85)
  line L15 (-24.05, 23.85) -> (-38.05, 23.85)
  line L16 (-19, 95) -> (-5, 95)
  line L17 (-5, 95) -> (-5, 81)
  line L18 (-5, 81) -> (-19, 81)
  line L19 (-19, 81) -> (-19, 95)
  line L20 (-38.05, 75.95) -> (-24.05, 75.95)
  line L21 (-24.05, 75.95) -> (-24.05, 61.95)
  line L22 (-24.05, 61.95) -> (-38.05, 61.95)
  line L23 (-38.05, 61.95) -> (-38.05, 75.95)
  line L24 (-19, 56.9) -> (-5, 56.9)
  line L25 (-5, 56.9) -> (-5, 42.9)
  line L26 (-5, 42.9) -> (-19, 42.9)
  line L27 (-19, 42.9) -> (-19, 56.9)
  line L28 (-19, 23.85) -> (-19, 37.85)
  line L29 (-19, 37.85) -> (-5, 37.85)
  line L30 (-5, 37.85) -> (-5, 23.85)
  line L31 (-5, 23.85) -> (-19, 23.85)
  line L32 (-38.05, 42.9) -> (-38.05, 56.9)
  line L33 (-38.05, 56.9) -> (-24.05, 56.9)
  line L34 (-24.05, 56.9) -> (-24.05, 42.9)
  line L35 (-24.05, 42.9) -> (-38.05, 42.9)
  line L36 (-66.9, 56.225) -> (-66.9, 85.865)
  line L37 (-66.9, 85.865) -> (-48.98, 85.865)
  line L38 (-48.98, 85.865) -> (-48.98, 56.225)
  line L39 (-48.98, 56.225) -> (-66.9, 56.225)
  arc A0 (-61.2435, 44.6) -> (-66.755, 39.0018) centre (-60.7672, 38.6189) ccw
  line L40 (-61.2435, 44.6) -> (-60.2909, 44.6)
  arc A1 (-66.755, 38.2361) -> (-60.2909, 44.6) centre (-60.7672, 38.6189) ccw
  line L41 (-66.755, 38.2361) -> (-66.755, 39.0018)
  circle A2 centre (-2.9963, 21.8321) radius 1
  circle A3 centre (-3, 97) radius 1
  circle A4 centre (-78.15, 97.0036) radius 1
  line L42 (-77.15, 21.923) -> (-77.15, 21.777)
  arc A5 (-77.15, 21.923) -> (-77.15, 21.777) centre (-78.1473, 21.85) ccw
extrude "Extrude43" add sketch "Sketch27" sketch "Sketch24" against normal blind 2 contours A4 | L42 A5 of sketch 2 contours A7 | A9
sketch "Sketch28" plane through (0, 2, 0) normal (0, 1, 0) x (-1, 0, 0)
  line L0 (-81.15, 100.965) -> (-81.15, 17.885)
  line L1 (-81.15, 17.885) -> (0, 17.885)
  line L2 (0, 17.885) -> (0, 100.965)
  line L3 (0, 100.965) -> (-81.15, 100.965)
  line L4 (-38.05, 95) -> (-24.05, 95)
  line L5 (-24.05, 95) -> (-24.05, 81)
  line L6 (-24.05, 81) -> (-38.05, 81)
  line L7 (-38.05, 81) -> (-38.05, 95)
  line L8 (-19, 61.95) -> (-19, 75.95)
  line L9 (-19, 75.95) -> (-5, 75.95)
  line L10 (-5, 75.95) -> (-5, 61.95)
  line L11 (-5, 61.95) -> (-19, 61.95)
  line L12 (-38.05, 23.85) -> (-38.05, 37.85)
  line L13 (-38.05, 37.85) -> (-24.05, 37.85)
  line L14 (-24.05, 37.85) -> (-24.05, 23.85)
  line L15 (-24.05, 23.85) -> (-38.05, 23.85)
  line L16 (-19, 95) -> (-5, 95)
  line L17 (-5, 95) -> (-5, 81)
  line L18 (-5, 81) -> (-19, 81)
  line L19 (-19, 81) -> (-19, 95)
  line L20 (-38.05, 75.95) -> (-24.05, 75.95)
  line L21 (-24.05, 75.95) -> (-24.05, 61.95)
  line L22 (-24.05, 61.95) -> (-38.05, 61.95)
  line L23 (-38.05, 61.95) -> (-38.05, 75.95)
  line L24 (-19, 56.9) -> (-5, 56.9)
  line L25 (-5, 56.9) -> (-5, 42.9)
  line L26 (-5, 42.9) -> (-19, 42.9)
  line L27 (-19, 42.9) -> (-19, 56.9)
  line L28 (-19, 23.85) -> (-19, 37.85)
  line L29 (-19, 37.85) -> (-5, 37.85)
  line L30 (-5, 37.85) -> (-5, 23.85)
  line L31 (-5, 23.85) -> (-19, 23.85)
  line L32 (-38.05, 42.9) -> (-38.05, 56.9)
  line L33 (-38.05, 56.9) -> (-24.05, 56.9)
  line L34 (-24.05, 56.9) -> (-24.05, 42.9)
  line L35 (-24.05, 42.9) -> (-38.05, 42.9)
  line L36 (-66.9, 56.225) -> (-66.9, 85.865)
  line L37 (-66.9, 85.865) -> (-48.98, 85.865)
  line L38 (-48.98, 85.865) -> (-48.98, 56.225)
  line L39 (-48.98, 56.225) -> (-66.9, 56.225)
  arc A0 (-61.2435, 44.6) -> (-66.755, 39.0018) centre (-60.7672, 38.6189) ccw
  line L40 (-61.2435, 44.6) -> (-60.2909, 44.6)
  arc A1 (-66.755, 38.2361) -> (-60.2909, 44.6) centre (-60.7672, 38.6189) ccw
  line L41 (-66.755, 38.2361) -> (-66.755, 39.0018)
  line L42 (0, 17.885) -> (0, 20.885)
  line L43 (0, 20.885) -> (-3, 20.885)
  circle A2 centre (-3, 20.885) radius 1
  line L44 (0, 17.885) -> (0, 21.885)
  line L45 (0, 21.885) -> (-4, 21.885)
  circle A3 centre (-4, 21.885) radius 4
  line L46 (-81.15, 17.885) -> (-81.15, 20.885)
  line L47 (-81.15, 20.885) -> (-78.15, 20.885)
  circle A4 centre (-78.15, 20.885) radius 1
  line L48 (-81.15, 17.885) -> (-81.15, 21.885)
  line L49 (-81.15, 21.885) -> (-77.15, 21.885)
  circle A5 centre (-77.15, 21.885) radius 4
  line L50 (-81.15, 100.965) -> (-77.15, 100.965)
  line L51 (-77.15, 100.965) -> (-77.15, 96.965)
  line L52 (-81.15, 100.965) -> (-78.15, 100.965)
  line L53 (-78.15, 100.965) -> (-78.15, 97.965)
  circle A6 centre (-78.15, 97.965) radius 1
  circle A7 centre (-77.15, 96.965) radius 4
  line L54 (0, 100.965) -> (-3, 100.965)
  line L55 (-3, 100.965) -> (-3, 97.965)
  line L56 (0, 100.965) -> (-4, 100.965)
  line L57 (-4, 100.965) -> (-4, 96.965)
  circle A8 centre (-3, 97.965) radius 1
  circle A9 centre (-4, 96.965) radius 4
  dimension "d237" = 3
  dimension "d238" = 3
  dimension "d239" = 2
  dimension "d240" = 4
  dimension "d241" = 4
  dimension "d242" = 8
  dimension "d243" = 3
  dimension "d244" = 3
  dimension "d245" = 2
  dimension "d246" = 4
  dimension "d247" = 4
  dimension "d248" = 8
  dimension "d249" = 4
  dimension "d250" = 4
  dimension "d251" = 3
  dimension "d252" = 3
  dimension "d253" = 2
  dimension "d254" = 8
  dimension "d255" = 3
  dimension "d256" = 3
  dimension "d257" = 4
  dimension "d258" = 4
  dimension "d259" = 2
  dimension "d260" = 8
  constraint coincident L1.end L2.start
  constraint perpendicular L1 L42
  constraint perpendicular L42 L43
  constraint coincident L43.end A2.centre
  constraint perpendicular L1 L44
  constraint perpendicular L44 L45
  constraint coincident L45.end A3.centre
  constraint coincident L0.end L1.start
  constraint perpendicular L1 L46
  constraint perpendicular L46 L47
  constraint coincident L47.end A4.centre
  constraint perpendicular L47 L48
  constraint perpendicular L48 L49
  constraint coincident L49.end A5.centre
  constraint coincident L0.start L3.end
  constraint perpendicular L0 L50
  constraint perpendicular L50 L51
  constraint perpendicular L0 L52
  constraint perpendicular L52 L53
  constraint coincident L53.end A6.centre
  constraint coincident L51.end A7.centre
  constraint coincident L2.end L3.start
  constraint perpendicular L2 L54
  constraint perpendicular L54 L55
  constraint perpendicular L2 L56
  constraint perpendicular L3 L57
  constraint coincident L55.end A8.centre
  constraint coincident L57.end A9.centre
  measures "d237" distance of L1.end L42.end
  measures "d238" distance of L42.end L43.end
  measures "d239" diameter of A2
  measures "d240" distance of L1.end L44.end
  measures "d241" distance of L44.end L45.end
  measures "d242" diameter of A3
  measures "d243" distance of L0.end L46.end
  measures "d244" distance of L46.end L47.end
  measures "d245" diameter of A4
  measures "d246" distance of L0.end L48.end
  measures "d247" distance of L48.end L49.end
  measures "d248" diameter of A5
  measures "d249" distance of L0.start L50.end
  measures "d250" distance of L50.end L51.end
  measures "d251" distance of L0.start L52.end
  measures "d252" distance of L52.end L53.end
  measures "d253" diameter of A6
  measures "d254" diameter of A7
  measures "d255" distance of L2.end L54.end
  measures "d256" distance of L54.end L55.end
  measures "d257" distance of L2.end L56.end
  measures "d258" distance of L56.end L57.end
  measures "d259" diameter of A8
  measures "d260" diameter of A9
extrude "Extrude44" cut sketch "Sketch28" against normal blind 4 contours L0 L47 L48 A5 | L0 L1 L46 L47 L48 A5 | L0 L3 L50 L52 L53 A7 | A4 | L3 L50 L53 A7 | A6 | L1 L2 L42 L43 L44 A3 | L3 L55 L56 A9 | L2 L43 L44 A3 | L2 L3 L54 L55 L56 A9 | A8 | A2
extrude "Extrude45" add sketch "Sketch23" against normal blind 2 contours L4 L5 L6 L7 | L8 L9 L10 L11 | L12 L13 L14 L15 | L16 L17 L18 L19 | L20 L21 L22 L23 | L24 L25 L26 L27 | L28 L29 L30 L31 | L32 L33 L34 L35
delete_face "DeleteFace11" 1 faces at (0.5359, 0.6667, 98.965)
delete_face "DeleteFace12" 1 faces at (80.93, 0.6667, 98.2733)
delete_face "DeleteFace13" 1 faces at (77.1698, 0.6667, 98.1631)
delete_face "DeleteFace14" 1 faces at (2.0012, 0.6667, 98.0148)
delete_face "DeleteFace15" 1 faces at (2.0012, 0.6667, 20.8352)
delete_face "DeleteFace16" 1 faces at (78.5613, 1.3333, 21.7965)
delete_face "DeleteFace17" 1 faces at (0.22, 0.6667, 20.5767)
delete_face "DeleteFace18" 1 faces at (78.9829, 0.6667, 18.3297)
delete_face "DeleteFace19" 1 faces at (79.0098, -0.0019, 28.2309)
delete_face "DeleteFace20" 1 faces at (79.1958, -0.0019, 87.2109)
delete_face "DeleteFace21" 1 faces at (45.2721, -0.0091, 84.7389)
delete_face "DeleteFace22" 1 faces at (50.3256, -0.0019, 29.5356)
extrude "Extrude46" add 1 faces at (81.15, 0.6667, 73.2717) along direction (1, 0, 0) blind 2.5
extrude "Extrude47" cut 1 faces at (0, 0.6667, 73.2717) along direction (1, 0, 0) blind 2.5
fillet "Fillet3" radius 1 4 edges at (43.6039, 0, 30.879) (72.6127, 0, 30.849) (43.5539, 0, 89.909) (72.7988, 0, 89.829)